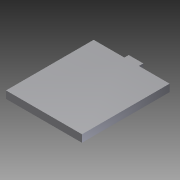
# Autodesk Inventor part: bateria
Saved by Autodesk Inventor 2012 (Build 160160000, 160)
## iProperties
Created: 2012-12-27
Part Number: bateria
Material: Default
Document SubType Name: Modeling
Designer: otrebor
Density: 1 g/cm^3
Author: otrebor
Autodesk Inventor part; units mm, degrees
ref_plane "YZ Plane" through (0, 0, 0) normal (1, 0, 0) x (0, 1, 0)
ref_plane "XZ Plane" through (0, 0, 0) normal (0, 1, 0) x (-1, 0, 0)
ref_plane "XY Plane" through (0, 0, 0) normal (0, 0, 1) x (1, 0, 0)
sketch "Boceto1" plane through (0, 0, 0) normal (0, 0, 1) x (1, 0, 0)
  line L0 (0, 0) -> (52, 0)
  line L1 (52, 0) -> (52, 60)
  line L2 (0, 60) -> (0, 0)
  line L3 (26, 63) -> (21, 63)
  line L4 (21, 63) -> (21, 60)
  line L5 (26, 63) -> (31, 63)
  line L6 (31, 63) -> (31, 60)
  line L7 (52, 60) -> (31, 60)
  line L8 (21, 60) -> (0, 60)
  dimension "d0" = 52
  dimension "d1" = 60
  constraints: 18 end point, 3 parallel, 3 perpendicular, 1 coincident, 1 horizontal
  measures "d0" distance of L0.start L0.end
  measures "d1" distance of L0.end L1.end
extrude "Extrusión1" add sketch "Boceto1" along normal blind 5
